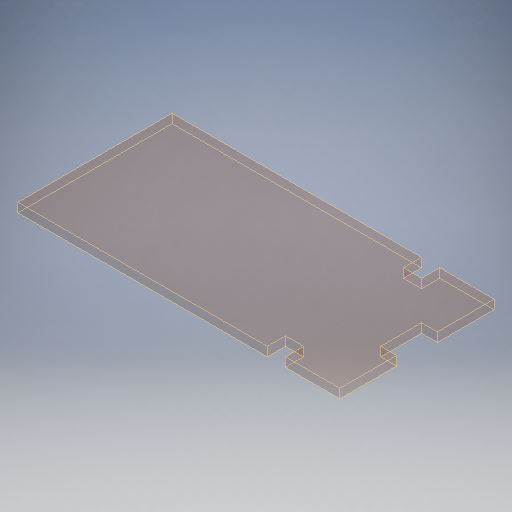
# Autodesk Inventor part: cowl_up
Saved by Autodesk Inventor 2025.2 (Build 292293000, 293)
## iProperties
Created: 2025-02-08
Part Number: cowl_up
Material: 폴리카보네이트, 흐릿
Document SubType Name: Modeling
Designer: jbhma
Density: 1.2 g/cm^3
Appearance: 폴리카보네이트 - 흐릿함
Author: jbhma
Autodesk Inventor part; units mm, degrees
ref_plane "YZ Plane" through (0, 0, 0) normal (1, 0, 0) x (0, 1, 0)
ref_plane "XZ Plane" through (0, 0, 0) normal (0, 1, 0) x (-1, 0, 0)
ref_plane "XY Plane" through (0, 0, 0) normal (0, 0, 1) x (1, 0, 0)
sketch "스케치1" plane through (0, 0, 0) normal (0, 1, 0) x (-1, 0, 0)
  line L0 (0, 0) -> (-710, 0)
  line L1 (-710, 0) -> (-710, -340)
  line L2 (-710, -340) -> (0, -340)
  line L3 (0, -340) -> (0, 0)
  line L4 (-710, -340) -> (-590, -340)
  line L5 (-710, -340) -> (-590, -340) construction
  line L6 (-590, -340) -> (-550, -340)
  line L7 (-550, -340) -> (-550, -300)
  line L8 (-550, -300) -> (-590, -300)
  line L9 (-590, -300) -> (-590, -340)
  line L10 (-710, 0) -> (-590, 0)
  line L11 (-710, 0) -> (-590, 0) construction
  line L12 (-590, 0) -> (-550, 0)
  line L13 (-550, 0) -> (-550, -40)
  line L14 (-550, -40) -> (-590, -40)
  line L15 (-590, -40) -> (-590, 0)
  line L16 (-710, 0) -> (-710, -170)
  line L17 (-710, 0) -> (-540, 0) construction
  line L18 (-710, -170) -> (-710, -125)
  line L19 (-710, -170) -> (-665, -170) construction
  line L20 (-710, -125) -> (-675, -125)
  line L21 (-675, -125) -> (-675, -215)
  line L22 (-675, -215) -> (-710, -215)
  line L23 (-710, -215) -> (-710, -125)
  dimension "d0" = 710
  dimension "d1" = 340
  dimension "d2" = 120
  dimension "d3" = 0
  dimension "d4" = 40
  dimension "d5" = 40
  dimension "d6" = 120
  dimension "d7" = 0
  dimension "d8" = 40
  dimension "d9" = 40
  dimension "d10" = 170
  dimension "d11" = 90
  dimension "d12" = 45
  dimension "d13" = 90
  dimension "d14" = 35
  dimension "d15" = 90
  constraints: 48 end point, 8 horizontal, 8 parallel, 4 collinear, 4 equal length, 4 perpendicular
  measures "d0" distance of L2.end L1.end
  measures "d1" distance of L1.end L0.end
  measures "d2" distance of L1.end L4.end
  measures "d3" distance between parallel lines of L4 L5
  measures "d4" distance of L8.end L7.end
  measures "d5" distance of L7.end L6.end
  measures "d6" distance of L0.end L10.end
  measures "d7" distance between parallel lines of L10 L11
  measures "d8" distance of L13.end L14.end
  measures "d9" distance of L12.end L13.end
  measures "d10" distance of L0.end L16.end
  measures "d11" angle of L16 L17
  measures "d12" distance of L16.end L18.end
  measures "d13" angle of L19 L18
  measures "d14" distance of L21.end L22.end
  measures "d15" distance of L20.end L21.end
extrude "돌출1" add sketch "스케치1" along normal blind 20 contours L3 L2 L7 L8 L9 L1 L22 L21 L20 L0 L15 L14 L13
